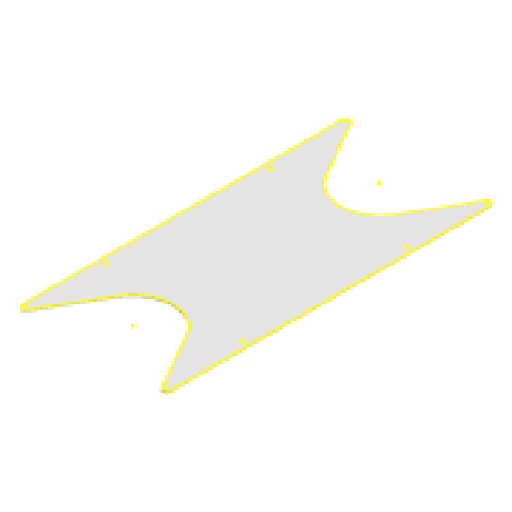
# Autodesk Inventor part: bottomPlate
Saved by Autodesk Inventor 2023 (Build 270158000, 158)
## iProperties
Created: 2022-10-10
Part Number: bottomPlate
Material: Generic
Document SubType Name: Modeling
Designer: deli
Density: 1 g/cm^3
Appearance: Default
Author: deli
Autodesk Inventor part; units mm, degrees
ref_plane "YZ Plane" through (0, 0, 0) normal (1, 0, 0) x (0, 1, 0)
ref_plane "XZ Plane" through (0, 0, 0) normal (0, 1, 0) x (-1, 0, 0)
ref_plane "XY Plane" through (0, 0, 0) normal (0, 0, 1) x (1, 0, 0)
sketch "Sketch1" plane through (0, 0, 0) normal (0, 1, 0) x (-1, 0, 0)
  arc A0 (-96, -365.415) -> (-86.6583, -367.8949) centre (-91, -365.415) ccw
  line L0 (-86.6583, -367.8949) -> (-44.0681, -293.3293)
  arc A1 (44.0681, -293.3293) -> (-44.0681, -293.3293) centre (0, -318.5) ccw
  line L1 (44.0681, -293.3293) -> (86.6583, -367.8949)
  arc A2 (86.6583, -367.8949) -> (96, -365.415) centre (91, -365.415) ccw
  line L2 (96, -365.415) -> (96, 46.915)
  arc A3 (96, 46.915) -> (86.6583, 49.3949) centre (91, 46.915) ccw
  line L3 (86.6583, 49.3949) -> (44.0681, -25.1707)
  arc A4 (-44.0681, -25.1707) -> (44.0681, -25.1707) centre (0, 0) ccw
  line L4 (-44.0681, -25.1707) -> (-86.6583, 49.3949)
  arc A5 (-86.6583, 49.3949) -> (-96, 46.915) centre (-91, 46.915) ccw
  line L5 (-96, 46.915) -> (-96, -365.415)
  circle A6 centre (-88, -53.3662) radius 2
  circle A7 centre (88, -53.3662) radius 2
  circle A8 centre (-88, -265.1338) radius 2
  circle A9 centre (88, -265.1338) radius 2
  point P0 (0, 0)
  point P1 (-86.6583, 49.3949)
  point P2 (-96, -365.415)
  point P3 (44.0681, -293.3293)
  point P4 (96, -365.415)
  point P5 (96, 46.915)
  constraints: 12 end point, 12 point on circle, 10 centre point
extrude "Extrusion1" add sketch "Sketch1" along normal blind 3.175
sketch "Sketch2" plane through (0, 3.175, 0) normal (0, 1, 0) x (1, 0, 0)
  arc A0 (86.6583, -49.3949) -> (96, -46.915) centre (91, -46.915) ccw projected
  line L0 (96, -46.915) -> (96, 365.415) projected
  arc A1 (96, 365.415) -> (86.6583, 367.8949) centre (91, 365.415) ccw projected
  line L1 (86.6583, 367.8949) -> (44.0681, 293.3293) projected
  arc A2 (-44.0681, 293.3293) -> (44.0681, 293.3293) centre (0, 318.5) ccw projected
  line L2 (-44.0681, 293.3293) -> (-86.6583, 367.8949) projected
  arc A3 (-86.6583, 367.8949) -> (-96, 365.415) centre (-91, 365.415) ccw projected
  line L3 (-96, 365.415) -> (-96, -46.915) projected
  arc A4 (-96, -46.915) -> (-86.6583, -49.3949) centre (-91, -46.915) ccw projected
  line L4 (-86.6583, -49.3949) -> (-44.0681, 25.1707) projected
  arc A5 (44.0681, 25.1707) -> (-44.0681, 25.1707) centre (0, 0) ccw projected
  line L5 (44.0681, 25.1707) -> (86.6583, -49.3949) projected
  circle A6 centre (-88, 265.1338) radius 2 projected
  circle A7 centre (88, 265.1338) radius 2 projected
  circle A8 centre (-88, 53.3662) radius 2 projected
  circle A9 centre (88, 53.3662) radius 2 projected
  point P0 (0, 0)
body "Solid1"
